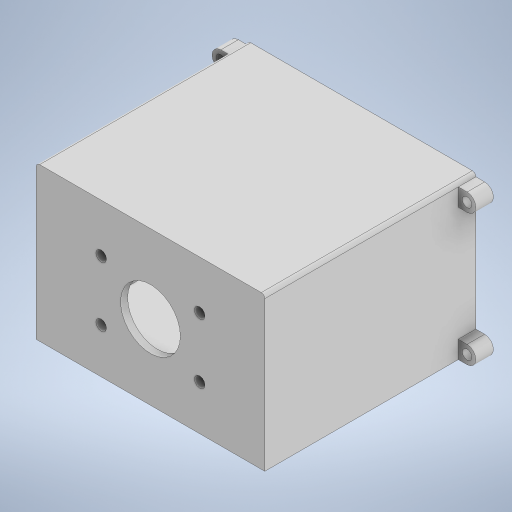
# Autodesk Inventor part: CAMCOVER
Saved by Autodesk Inventor 2023.1 (Build 271208000, 208)
## iProperties
Created: 2023-02-03
Part Number: CAMCOVER
Material: Generic
Document SubType Name: Modeling
Designer: liaar
Density: 1 g/cm^3
Appearance: Default
Author: liaar
Autodesk Inventor part; units mm, degrees
ref_plane "YZ Plane" through (0, 0, 0) normal (1, 0, 0) x (0, 1, 0)
ref_plane "XZ Plane" through (0, 0, 0) normal (0, 1, 0) x (-1, 0, 0)
sketch "Sketch1" plane through (0, 0, 0) normal (0, 0, 1) x (1, 0, 0)
  line L0 (0, 0) -> (-65, 0)
  line L1 (-65, 0) -> (-65, 43.5)
  line L2 (-65, 43.5) -> (0, 43.5)
  line L3 (0, 43.5) -> (0, 0)
  dimension "d0" = 43.5
  dimension "d1" = 65
  constraints: 8 end point, 2 parallel, 1 horizontal, 1 perpendicular
  measures "d0" distance of L2.end L0.start
  measures "d1" distance of L1.end L2.end
extrude "Extrusion1" add sketch "Sketch1" along normal blind 60
sketch "Sketch2" plane through (0, 0, 0) normal (0, 0, -1) x (-1, 0, 0)
  line L0 (1.8, 41.7) -> (63.2, 41.7)
  line L1 (63.2, 41.7) -> (63.2, 1.8)
  line L2 (63.2, 1.8) -> (1.8, 1.8)
  line L3 (1.8, 1.8) -> (1.8, 41.7)
  line L4 (65, 43.5) -> (65, 0) projected
  line L5 (0, 43.5) -> (65, 43.5) projected
  line L6 (0, 0) -> (0, 43.5) projected
  line L7 (65, 0) -> (0, 0) projected
  point P0 (65, 21.75)
  dimension "d4" = 1.8
  dimension "d5" = 1.8
  dimension "d6" = 1.8
  dimension "d7" = 1.8
  constraints: 8 end point, 2 parallel, 1 horizontal, 1 midpoint, 1 perpendicular
  measures "d4" distance from line of point (65, 21.75) L1
  measures "d5" distance between parallel lines of L5 L0
  measures "d6" distance between parallel lines of L6 L3
  measures "d7" distance between parallel lines of L7 L2
extrude "Extrusion2" cut sketch "Sketch2" against normal blind 58 contours L0 L1 L2 L3
fillet "Fillet1" radius 1 2 edges at (-65, 43.5, 30) (0, 43.5, 30)
sketch "Sketch5" plane through (0, 0, 60) normal (0, 0, 1) x (1, 0, 0)
  circle A0 centre (-32.5, 21.25) radius 8.5
  line L0 (-1, 43.5) -> (-64, 43.5) projected
  line L1 (-65, 42.5) -> (-65, 0) projected
  point P0 (0, 0)
  point P1 (-32.5, 43.5)
  point P2 (-65, 21.25)
  dimension "d41" = 17
  constraints: 2 midpoint, 1 centre point, 1 horizontal alignment, 1 vertical alignment
  measures "d41" diameter of A0
extrude "Extrusion5" cut sketch "Sketch5" against normal blind 10
sketch "Sketch6" plane through (0, 0, 60) normal (0, 0, 1) x (1, 0, 0)
  line L0 (-47.5, 33.25) -> (-17.5, 33.25)
  line L1 (-17.5, 33.25) -> (-17.5, 9.25)
  line L2 (-17.5, 9.25) -> (-47.5, 9.25)
  line L3 (-47.5, 9.25) -> (-47.5, 33.25)
  line L4 (-1, 43.5) -> (-64, 43.5) projected
  line L5 (0, 0) -> (0, 42.5) projected
  circle A0 centre (-44.5, 32.25) radius 1.5
  circle A1 centre (-46.5, 29.75) radius 1.5
  line L6 (-32.5, 33.25) -> (-32.5, 9.25) construction
  line L7 (-47.5, 21.25) -> (-17.5, 21.25) construction
  line L8 (-17.5, 33.25) -> (-47.5, 33.25)
  line L9 (-17.5, 9.25) -> (-17.5, 33.25)
  circle A2 centre (-20.5, 32.25) radius 1.5
  circle A3 centre (-18.5, 29.75) radius 1.5
  circle A4 centre (-44.5, 10.25) radius 1.5
  circle A5 centre (-46.5, 12.75) radius 1.5
  circle A6 centre (-18.5, 12.75) radius 1.5
  circle A7 centre (-20.5, 10.25) radius 1.5
  point P0 (-32.5, 43.5)
  point P1 (0, 21.25)
  point P2 (-47.5, 9.25)
  point P3 (-17.5, 9.25)
  point P4 (-17.5, 9.25)
  point P5 (-47.5, 9.25)
  dimension "d44" = 30
  dimension "d45" = 24
  dimension "d46" = 3
  dimension "d47" = 3
  dimension "d49" = 1
  dimension "d50" = 1
  dimension "d53" = 8.5
  dimension "d54" = 12
  constraints: 16 end point, 12 symmetric about line, 8 centre point, 6 midpoint, 2 horizontal, 2 parallel, 1 horizontal alignment, 1 perpendicular, 1 vertical alignment, 6 other
  measures "d44" distance of L0.start L0.end
  measures "d45" distance of L0.end L1.end
  measures "d46" diameter of A0
  measures "d47" diameter of A1
  measures "d49" distance from line of L0 A0.centre
  measures "d50" distance from line of L3 A1.centre
  measures "d53" distance from line of L7 A1.centre
  measures "d54" distance from line of L6 A0.centre
extrude "Extrusion6" cut sketch "Sketch6" against normal up to surface (2 mm away) contours A1 L3 | L3 A1 | A5 L3 | L3 A5 | A3 L1 | L1 A3 | A6 L1 | L1 A6
sketch "Sketch7" plane through (0, 0, 60) normal (0, 0, 1) x (1, 0, 0)
  line L0 (-65, 42.5) -> (-65, 0) projected
  line L1 (-65, 42.5) -> (-70, 42.5)
  line L2 (-70, 42.5) -> (-70, 37.5)
  line L3 (-70, 37.5) -> (-65, 37.5)
  line L4 (-65, 37.5) -> (-65, 42.5)
  line L5 (0, 0) -> (0, 42.5) projected
  line L6 (0, 42.5) -> (5, 42.5)
  line L7 (5, 42.5) -> (5, 37.5)
  line L8 (5, 37.5) -> (0, 37.5)
  line L9 (0, 37.5) -> (0, 42.5)
  line L10 (-65, 0) -> (0, 0) projected
  line L11 (0, 0) -> (5, 0)
  line L12 (5, 0) -> (5, 5)
  line L13 (5, 5) -> (0, 5)
  line L14 (0, 5) -> (0, 0)
  line L15 (-65, 0) -> (-70, 0)
  line L16 (-70, 0) -> (-70, 5)
  line L17 (-70, 5) -> (-65, 5)
  line L18 (-65, 5) -> (-65, 0)
  circle A0 centre (-67.5, 40) radius 1.35
  circle A1 centre (-67.5, 2.5) radius 1.35
  circle A2 centre (2.5, 2.5) radius 1.35
  circle A3 centre (2.5, 40) radius 1.35
  dimension "d57" = 5
  dimension "d58" = 5
  dimension "d59" = 5
  dimension "d60" = 5
  dimension "d61" = 5
  dimension "d62" = 5
  dimension "d63" = 5
  dimension "d64" = 5
  dimension "d65" = 2.7
  dimension "d66" = 2.7
  dimension "d67" = 2.7
  dimension "d68" = 2.7
  dimension "d69" = 2.5
  dimension "d70" = 2.5
  dimension "d71" = 2.5
  dimension "d72" = 2.5
  dimension "d73" = 2.5
  dimension "d74" = 2.5
  dimension "d75" = 2.5
  dimension "d76" = 2.5
  constraints: 32 end point, 8 parallel, 4 centre point, 4 horizontal, 4 perpendicular
  measures "d57" distance of L0.start L1.end
  measures "d58" distance of L1.end L2.end
  measures "d59" distance of L15.end L16.end
  measures "d60" distance of L16.end L17.end
  measures "d61" distance of L12.end L13.end
  measures "d62" distance of L11.end L12.end
  measures "d63" distance of L5.end L6.end
  measures "d64" distance of L6.end L7.end
  measures "d65" diameter of A3
  measures "d66" diameter of A2
  measures "d67" diameter of A1
  measures "d68" diameter of A0
  measures "d69" distance from line of L1 A0.centre
  measures "d70" distance from line of L2 A0.centre
  measures "d71" distance from line of L16 A1.centre
  measures "d72" distance from line of L17 A1.centre
  measures "d73" distance from line of L13 A2.centre
  measures "d74" distance from line of L14 A2.centre
  measures "d75" distance from line of L5 A3.centre
  measures "d76" distance from line of L6 A3.centre
ref_plane "Work Plane1" through (-65, 43.5, 0) normal (0, 0, 1) x (0, -1, 0)
sketch "Sketch8" plane through (-65, 43.5, 0) normal (0, 0, 1) x (0, -1, 0)
  line L0 (6, 70) -> (6, 65) projected
  circle A0 centre (3.5, 67.5) radius 1.35 projected
  line L1 (1, 70) -> (6, 70) projected
  line L2 (1, 65) -> (1, 70) projected
  line L3 (43.5, 65) -> (43.5, 70) projected
  circle A1 centre (41, 67.5) radius 1.35 projected
  line L4 (43.5, 70) -> (38.5, 70) projected
  line L5 (38.5, 70) -> (38.5, 65) projected
  line L6 (43.5, 0) -> (43.5, -5) projected
  circle A2 centre (41, -2.5) radius 1.35 projected
  line L7 (43.5, -5) -> (38.5, -5) projected
  line L8 (38.5, -5) -> (38.5, 0) projected
  line L9 (6, -5) -> (6, 0) projected
  circle A3 centre (3.5, -2.5) radius 1.35 projected
  line L10 (1, -5) -> (6, -5) projected
  line L11 (1, 0) -> (1, -5) projected
  circle A4 centre (3.5, 67.5) radius 1.35
  circle A5 centre (41, 67.5) radius 1.35
  circle A6 centre (41, -2.5) radius 1.35
  circle A7 centre (3.5, -2.5) radius 1.35
  line L12 (1, 0) -> (43.5, 0) projected
  line L13 (1, 0) -> (6, 0)
  line L14 (6, 0) -> (6, -5)
  line L15 (6, -5) -> (1, -5)
  line L16 (1, -5) -> (1, 0)
  line L17 (38.5, 0) -> (43.5, 0)
  line L18 (43.5, 0) -> (43.5, -5)
  line L19 (43.5, -5) -> (38.5, -5)
  line L20 (38.5, -5) -> (38.5, 0)
  line L21 (38.5, 65) -> (43.5, 65)
  line L22 (43.5, 65) -> (43.5, 70)
  line L23 (43.5, 70) -> (38.5, 70)
  line L24 (38.5, 70) -> (38.5, 65)
  line L25 (43.5, 65) -> (1, 65) projected
  line L26 (1, 65) -> (6, 65)
  line L27 (6, 65) -> (6, 70)
  line L28 (6, 70) -> (1, 70)
  line L29 (1, 70) -> (1, 65)
  constraints: 32 end point, 8 parallel, 4 centre point, 4 coincident, 4 concentric, 4 horizontal, 4 perpendicular
extrude "Extrusion7" add sketch "Sketch8" along normal blind 5
full round fillet "Full Round Fillet5" first side at (-66.6667, 42.5, 1.6667) centre faces at (-70, 40.8333, 1.6667) second side at (-68.3333, 37.5, 1.6667)
full round fillet "Full Round Fillet6" first side at (-43.3333, 0, 23.3333) centre faces at (-70, 3.3333, 1.6667) second side at (-66.6667, 5, 1.6667)
full round fillet "Full Round Fillet7" first side at (1.6667, 42.5, 3.3333) centre faces at (5, 39.1667, 1.6667) second side at (1.6667, 37.5, 1.6667)
full round fillet "Full Round Fillet8" first side at (-43.3333, 0, 23.3333) centre faces at (5, 1.6667, 1.6667) second side at (3.3333, 5, 1.6667)
body "Solid1"
